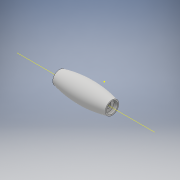
# Autodesk Inventor part: roller test
Saved by Autodesk Inventor 2018 (Build 220112000, 112)
## iProperties
Created: 2017-09-19
Part Number: roller test
Material: Generic
Document SubType Name: Modeling
Designer: M227958
Density: 1 g/cm^3
Appearance: Default
Author: M227958
Autodesk Inventor part; units mm, degrees
ref_plane "YZ Plane" through (0, 0, 0) normal (1, 0, 0) x (0, 1, 0)
ref_plane "XZ Plane" through (0, 0, 0) normal (0, 1, 0) x (-1, 0, 0)
ref_plane "Work Plane1" through (0, 0, 0) normal (0, -0.866, 0.5) x (1, 0, 0)
sketch "Sketch1" plane through (0, 0, 0) normal (0, -0.866, 0.5) x (1, 0, 0)
  circle A0 centre (0, 0) radius 97 construction
  dimension "d1" = 194
  constraints: 1 centre point, 1 coincident
  measures "d1" diameter of A0
sketch "Sketch2" plane through (0, 0, 0) normal (0, 1, 0) x (-1, 0, 0)
  point P0 (0, 0)
sketch "Sketch3" plane through (0, 0, 0) normal (0, 0, 1) x (1, 0, 0)
  ellipse E0 centre (0, 0) end of major axis (97, 0) minor radius 48.5 construction
  circle A0 centre (0, -31.5) radius 17
  line L0 (0, -31.5) -> (44.8665, -31.5)
  line L1 (0, -43) -> (44.8665, -43) construction
  line L2 (0, -31.5) -> (-44.8665, -31.5)
  line L3 (0, -43) -> (-44.8665, -43) construction
  line L4 (44.8665, -43) -> (44.8665, -31.5)
  line L5 (-44.8665, -43) -> (-44.8665, -31.5)
  arc A1 (-44.8665, -43) -> (44.8665, -43) centre (0, 137.25) ccw
  dimension "d3" = 11.5
  constraints: 12 end point, 4 horizontal, 2 centre point, 2 perpendicular, 2 point on circle, 4 other
  measures "d3" distance of L0.start L1.start
revolve "Revolution1" add sketch "Sketch3" angle 360 about axis through (0, -31.5, 0) along (1, 0, 0) picked at (1.261, -42.6913) contours L0 L4 A1 A0 | A0 L2 L0 | A0 A1 L5 L2
sketch "Sketch4" plane through (-44.8665, -31.5, 0) normal (-1, 0, 0) x (0, 0, 1)
  circle A0 centre (0, 0) radius 9.5
  point P0 (0, 31.5)
  dimension "d5" = 19
  constraints: 1 centre point
  measures "d5" diameter of A0
extrude "Extrusion1" cut sketch "Sketch4" against normal blind 6
sketch "Sketch5" plane through (-38.8665, -31.5, 0) normal (-1, 0, 0) x (0, 0, 1)
  circle A0 centre (0, 0) radius 4
  point P0 (0, 31.5)
  dimension "d8" = 8
  constraints: 1 centre point
  measures "d8" diameter of A0
extrude "Extrusion2" cut sketch "Sketch5" against normal blind 100
sketch "Sketch6" plane through (44.8665, -31.5, 0) normal (1, 0, 0) x (0, 0, -1)
  circle A0 centre (0, 0) radius 4 projected
  circle A1 centre (0, 0) radius 9.5
  point P0 (0, 31.5)
  constraints: 1 centre point, 1 coincident
extrude "Extrusion3" cut sketch "Sketch6" against normal blind 6
body "Solid1"
